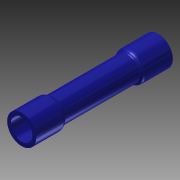
# Autodesk Inventor part: 22-18 double sided female tube red
Saved by Autodesk Inventor 2014 (Build 180170000, 170)
## iProperties
Created: 2013-07-20
Part Number: 22-18 double sided female tube red
Material: Generic
Document SubType Name: Modeling
Designer: Saville
Mass: 0.264175 g
Surface Area: 9.25104 cm^2
Volume: 0.264175 cm^3
Density: 1 g/cm^3
Appearance: Default
Author: Saville
Autodesk Inventor part; units mm, degrees
ref_plane "YZ Plane" through (0, 0, 0) normal (1, 0, 0) x (0, 1, 0)
ref_plane "XZ Plane" through (0, 0, 0) normal (0, 1, 0) x (-1, 0, 0)
ref_plane "XY Plane" through (0, 0, 0) normal (0, 0, 1) x (1, 0, 0)
sketch "Sketch1" plane through (0, 0, 0) normal (0, 0, 1) x (1, 0, 0)
  circle A0 centre (0, 0) radius 2.2225
  dimension "d0" = 4.445
  constraints: 1 centre point, 1 coincident
  measures "d0" diameter of A0
extrude "Extrusion1" add sketch "Sketch1" along normal mid plane 24.7269
sketch "Sketch2" plane through (0, 0, 12.36345) normal (0, 0, 1) x (1, 0, 0)
  circle A0 centre (0, 0) radius 2.2225 projected
  circle A1 centre (0, 0) radius 2.6289
  dimension "d3" = 5.2578
  constraints: 1 centre point, 1 coincident
  measures "d3" diameter of A1
extrude "Extrusion2" add sketch "Sketch2" against normal blind 5.461
fillet "Fillet1" radius 0.254 1 edges at (-2.2225, 0, 6.9024)
fillet "Fillet2" radius 0.762 1 edges at (-2.6289, 0, 6.9024)
mirror "Mirror1" about plane through (0, 0, 0) normal (0, 0, 1) of "Extrusion2", "Fillet1", "Fillet2"
shell "Shell1" thickness 0.6731 removed faces 2 at (-0.850836, 0.209712, -12.36345) at (-0.850836, 0.209712, 12.36345)
sketch "Sketch3" plane through (0, 0, 0) normal (1, 0, 0) x (0, 1, 0)
  line L0 (-2.6289, 7.46125) -> (-2.6289, 12.36345)
  line L1 (-2.6289, 12.36345) -> (-1.9558, 12.36345)
  line L2 (-1.9558, 12.36345) -> (-1.9558, 7.46125)
  line L3 (-1.5494, 6.64845) -> (-1.5494, -6.64845)
  line L4 (-1.9558, -7.46125) -> (-1.9558, -12.36345)
  line L5 (-1.9558, -12.36345) -> (-2.6289, -12.36345)
  line L6 (-2.6289, -12.36345) -> (-2.6289, -7.46125)
  arc A0 (-2.3241, -6.85165) -> (-2.2225, -6.64845) centre (-2.4765, -6.64845) ccw
  line L7 (-2.2225, -6.64845) -> (-2.2225, 6.64845)
  arc A1 (-2.2225, 6.64845) -> (-2.3241, 6.85165) centre (-2.4765, 6.64845) ccw
  arc A2 (2.3241, 6.85165) -> (2.2225, 6.64845) centre (2.4765, 6.64845) ccw
  line L8 (2.2225, 6.64845) -> (2.2225, -6.64845)
  arc A3 (2.2225, -6.64845) -> (2.3241, -6.85165) centre (2.4765, -6.64845) ccw
  line L9 (2.6289, -7.46125) -> (2.6289, -12.36345)
  line L10 (2.6289, -12.36345) -> (1.9558, -12.36345)
  line L11 (1.9558, -12.36345) -> (1.9558, -7.46125)
  line L12 (1.5494, -6.64845) -> (1.5494, 6.64845)
  line L13 (1.9558, 7.46125) -> (1.9558, 12.36345)
  line L14 (1.9558, 12.36345) -> (2.6289, 12.36345)
  line L15 (2.6289, 12.36345) -> (2.6289, 7.46125)
  line L16 (-1.5494, -7.41045) -> (-1.1811, -7.41045)
  line L17 (-1.1811, -7.41045) -> (-1.1811, 7.41045)
  line L18 (-1.1811, 7.41045) -> (-1.5494, 7.41045)
  line L19 (-1.5494, 7.41045) -> (-1.5494, -7.41045)
  line L20 (0, -17.30883) -> (0, 17.30883)
  arc A4 (-2.6289, 7.46125) -> (-2.3241, 6.85165) centre (-1.8669, 7.46125) ccw
  arc A5 (-1.9558, 7.46125) -> (-1.92024, 7.39013) centre (-1.8669, 7.46125) ccw
  arc A6 (-1.5494, 6.64845) -> (-1.92024, 7.39013) centre (-2.4765, 6.64845) ccw
  arc A7 (-1.92024, -7.39013) -> (-1.5494, -6.64845) centre (-2.4765, -6.64845) ccw
  arc A8 (-1.92024, -7.39013) -> (-1.9558, -7.46125) centre (-1.8669, -7.46125) ccw
  arc A9 (-2.3241, -6.85165) -> (-2.6289, -7.46125) centre (-1.8669, -7.46125) ccw
  arc A10 (2.3241, 6.85165) -> (2.6289, 7.46125) centre (1.8669, 7.46125) ccw
  arc A11 (2.6289, -7.46125) -> (2.3241, -6.85165) centre (1.8669, -7.46125) ccw
  arc A12 (1.9558, -7.46125) -> (1.92024, -7.39013) centre (1.8669, -7.46125) ccw
  arc A13 (1.5494, -6.64845) -> (1.92024, -7.39013) centre (2.4765, -6.64845) ccw
  arc A14 (1.92024, 7.39013) -> (1.5494, 6.64845) centre (2.4765, 6.64845) ccw
  arc A15 (1.92024, 7.39013) -> (1.9558, 7.46125) centre (1.8669, 7.46125) ccw
  point P0 (0, 0)
  dimension "d9" = 0.3683
  dimension "d10" = 0.762
  dimension "d11" = 0.762
  constraints: 8 end point, 2 parallel, 1 collinear, 1 horizontal, 1 perpendicular
  measures "d9" distance between parallel lines of L17 L19
  measures "d10" distance from line of L3.end L16
  measures "d11" distance from line of L18 L3.start
revolve "Revolution1" add sketch "Sketch3" angle 360 about axis through (0, 0, -10) along (0, 0, 1) separate body contours L19 L18 L17 L16 L3
chamfer "Chamfer1" distance 0.2032 angle 45 2 edges at (0, 1.1811, 7.4105) (0, 1.1811, -7.4105)
body "Solid1"
body "Solid2"
